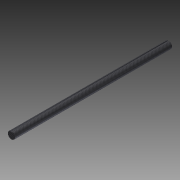
# Autodesk Inventor part: 11in axle
Saved by Autodesk Inventor 2011 SP1 (Build 150282100, 282)
## iProperties
Created: 2012-01-20
Part Number: 11in axle
Document SubType Name: Modeling
Designer: Christopher
Density: 1 g/cm^3
Author: Christopher
Autodesk Inventor part; units mm, degrees
ref_plane "YZ Plane" through (0, 0, 0) normal (1, 0, 0) x (0, 1, 0)
ref_plane "XZ Plane" through (0, 0, 0) normal (0, 1, 0) x (-1, 0, 0)
ref_plane "XY Plane" through (0, 0, 0) normal (0, 0, 1) x (1, 0, 0)
sketch "Sketch1" plane through (0, 0, 0) normal (0, 0, 1) x (1, 0, 0)
  circle A0 centre (0, 0) radius 6.35
  line L0 (-1.5875, 7.9375) -> (1.5875, 7.9375)
  line L1 (1.5875, 7.9375) -> (1.5875, 4.7625)
  line L2 (1.5875, 4.7625) -> (-1.5875, 4.7625)
  line L3 (-1.5875, 4.7625) -> (-1.5875, 7.9375)
  line L4 (1.5875, 4.7625) -> (1.5875, 6.1484)
  line L5 (-1.5875, 4.7625) -> (-1.5875, 6.1484)
  line L6 (1.5875, 4.7625) -> (-1.5875, 4.7625)
  point P0 (0, 4.7625)
  dimension "d0" = 12.7
  dimension "d1" = 3.175
  dimension "d2" = 3.175
  dimension "d3" = 4.7625
  constraints: 14 end point, 3 equal length, 2 point on circle, 2 point on line, 1 centre point, 1 coincident, 1 horizontal, 1 midpoint, 1 perpendicular, 1 vertical alignment
  measures "d0" diameter of A0
  measures "d1" distance of L0.end L1.end
  measures "d2" distance of L0.start L0.end
  measures "d3" distance from line of point (0, 0) L2
extrude "Extrusion1" add sketch "Sketch1" against normal blind 279.4 contours A0 L3 L2 L1 picked at (0.1781, 1.0658)
body "Solid1"
